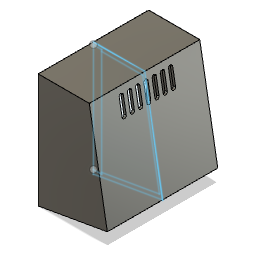
TrafficLight (Autodesk Fusion 360 archive; units mm, degrees)
design "PraxisAmpel2"
Autodesk Fusion 360 part; units mm, degrees
sketch "Sketch1" plane through (0, 0, 0) normal (0, 0, 1) x (1, 0, 0)
  line L0 (7.1104, -4.3777) -> (49.1586, 3.0365)
  line L1 (49.1586, 3.0365) -> (38.1927, 65.227)
  line L2 (38.1927, 65.227) -> (7.1104, 65.227)
  line L3 (7.1104, 65.227) -> (7.1104, -4.3777)
  line L4 (7.1104, 63.727) -> (12.1104, 63.727)
  line L5 (12.1104, 63.727) -> (12.1104, -1.973)
  line L6 (12.1104, -1.973) -> (7.1104, -1.973)
  line L7 (12.1104, 62.727) -> (37.1104, 62.727)
  line L8 (37.1104, 62.727) -> (47.2499, 5.2231)
  line L9 (47.2499, 5.2231) -> (12.1104, -0.973)
  dimension "d5" = 80
  dimension "d6" = 1.5
  dimension "d8" = 5
  dimension "d9" = 65.7
  dimension "d11" = 1.5
  dimension "d12" = 1
  dimension "d13" = 1
  dimension "d40" = 1.5
  dimension "d41" = 30
  constraint horizontal L2
  constraint vertical L3
  constraint perpendicular L0 L1
  constraint horizontal L4
  constraint vertical L5
  constraint horizontal L6
  constraint coincident L3 L4.start
  constraint coincident L5 L7.start
  constraint perpendicular L5 L7
  constraint parallel L1 L8
  constraint coincident L5 L9.end
  constraint parallel L0 L9
  measures "d5" angle of L0 L3
  measures "d6" distance of L2 L4
  measures "d8" distance of L3 L5
  measures "d9" distance of L4 L6
  measures "d11" distance of L0 L5.end
  measures "d12" distance of L5.end L9.end
  measures "d13" distance of L4.end L7.start
  measures "d40" distance of L1 L8
  measures "d41" horizontal distance of L4.start L7.end
extrude "Extrude4" add sketch "Sketch1" against normal blind 32.1 contours L3 L4 L5 L6 | L5 L7 L8 L9 makes body 1
extrude "Extrude3" add sketch "Sketch1" along normal blind 32.1 separate body contours L3 L4 L5 L6 | L5 L7 L8 L9 makes body 2
extrude "Extrude1" add sketch "Sketch1" along normal blind 33.6 separate body makes body 3
extrude "Extrude2" add 1 faces at (31.4873, 22.0968, 0) along direction (0, 0, -1) blind 33.6 on bodies 3 bodies 3
combine "Combine1" operation add target body 1 tool bodies 2
combine "Combine2" operation cut target body 3 tool bodies 1
sketch "Sketch2" plane through (0, 0, -33.6) normal (0, 0, -1) x (-1, 0, 0)
  line L0 (-7.1104, -4.3777) -> (-7.1104, 65.227)
  line L1 (-7.1104, 65.227) -> (-38.1927, 65.227)
  line L2 (-38.1927, 65.227) -> (-49.1586, 3.0365)
  line L3 (-49.1586, 3.0365) -> (-7.1104, -4.3777)
  line L4 (-7.1104, 8.6223) -> (-15.1104, 8.6223)
  line L5 (-17.1104, 6.6223) -> (-17.1104, 5.6223)
  line L6 (-15.1104, 3.6223) -> (-7.1104, 3.6223)
  arc A0 (-15.1104, 8.6223) -> (-17.1104, 6.6223) centre (-15.1104, 6.6223) ccw
  arc A1 (-17.1104, 5.6223) -> (-15.1104, 3.6223) centre (-15.1104, 5.6223) ccw
  line L7 (-7.1104, 65.227) -> (-7.1104, -4.3777)
  dimension "d23" = 2
  dimension "d24" = 2
  dimension "d26" = 8
  dimension "d27" = 10
  dimension "d28" = 5
  constraint coincident L0 L4.start
  constraint perpendicular L0 L4
  constraint perpendicular L4 L5
  constraint perpendicular L0 L6
  constraint tangent L4 A0
  constraint tangent L5 A0
  constraint tangent L5 A1
  constraint tangent L6 A1
  measures "d23" radius of A0
  measures "d24" radius of A1
  measures "d26" distance of L0.start L6
  measures "d27" distance of L5 L7
  measures "d28" distance of L4 L6
extrude "Extrude5" cut sketch "Sketch2" against normal blind 1.5 contours L0 L4 L5 L6 A0 A1 L7 bodies 3
sketch "Sketch3" plane through (48.1956, 8.4982, 0) normal (0.984808, 0.173648, 0) x (0, 0, -1)
  line L0 (33.6, 57.604) -> (-33.6, 57.604)
  line L1 (-33.6, 57.604) -> (-33.6, -5.546)
  line L2 (-33.6, -5.546) -> (33.6, -5.546)
  line L3 (33.6, -5.546) -> (33.6, 57.604)
  line L4 (1.25, 42.604) -> (1.25, 52.604)
  arc A0 (1.25, 52.604) -> (-1.25, 52.604) centre (0, 52.604) ccw
  line L5 (-1.25, 52.604) -> (-1.25, 42.604)
  arc A1 (-1.25, 42.604) -> (1.25, 42.604) centre (0, 42.604) ccw
  line L6 (0, 42.604) -> (0, 52.604) construction
  line L7 (0, 57.604) -> (0, 47.604) construction
  arc A2 (-13.75, 52.604) -> (-16.25, 52.604) centre (-15, 52.604) ccw
  arc A3 (-16.25, 42.604) -> (-13.75, 42.604) centre (-15, 42.604) ccw
  line L8 (-13.75, 42.604) -> (-13.75, 52.604)
  line L9 (-16.25, 52.604) -> (-16.25, 42.604)
  arc A4 (-8.75, 52.604) -> (-11.25, 52.604) centre (-10, 52.604) ccw
  arc A5 (-11.25, 42.604) -> (-8.75, 42.604) centre (-10, 42.604) ccw
  line L10 (-8.75, 42.604) -> (-8.75, 52.604)
  line L11 (-11.25, 52.604) -> (-11.25, 42.604)
  arc A6 (-3.75, 52.604) -> (-6.25, 52.604) centre (-5, 52.604) ccw
  arc A7 (-6.25, 42.604) -> (-3.75, 42.604) centre (-5, 42.604) ccw
  line L12 (-3.75, 42.604) -> (-3.75, 52.604)
  line L13 (-6.25, 52.604) -> (-6.25, 42.604)
  arc A8 (6.25, 52.604) -> (3.75, 52.604) centre (5, 52.604) ccw
  arc A9 (3.75, 42.604) -> (6.25, 42.604) centre (5, 42.604) ccw
  line L14 (6.25, 42.604) -> (6.25, 52.604)
  line L15 (3.75, 52.604) -> (3.75, 42.604)
  arc A10 (11.25, 52.604) -> (8.75, 52.604) centre (10, 52.604) ccw
  arc A11 (8.75, 42.604) -> (11.25, 42.604) centre (10, 42.604) ccw
  line L16 (11.25, 42.604) -> (11.25, 52.604)
  line L17 (8.75, 52.604) -> (8.75, 42.604)
  arc A12 (16.25, 52.604) -> (13.75, 52.604) centre (15, 52.604) ccw
  arc A13 (13.75, 42.604) -> (16.25, 42.604) centre (15, 42.604) ccw
  line L18 (16.25, 42.604) -> (16.25, 52.604)
  line L19 (13.75, 52.604) -> (13.75, 42.604)
  point P0 (0, 47.604)
  dimension "d31" = 2.5
  dimension "d32" = 10
  dimension "d33" = 10
  dimension "d36" = 5
  dimension "d37" = 0
  constraint tangent L4 A0
  constraint tangent A0 L5
  constraint parallel L4 L5
  constraint tangent L5 A1
  constraint tangent L4 A1
  constraint vertical L6
  constraint midpoint L6 P0
  constraint midpoint L0 L7.start
  constraint perpendicular L0 L7
  constraint coincident P0 L7.end
  measures "d31" diameter of A0
  measures "d32" distance of A1.centre A0.centre
  measures "d33" distance of L7.start P0
extrude "Extrude6" cut sketch "Sketch3" against normal blind 1.5 contours L4 A0 L5 A1 | A2 A3 L8 L9 | A4 A5 L10 L11 | A6 A7 L12 L13 | A8 A9 L14 L15 | A10 A11 L16 L17 | A12 A13 L18 L19 bodies 3
equation "wall_thickness = 1.5 mm"
equation "d6 = wall_thickness"
equation "d9 = 64.2 mm + wall_thickness"
equation "d11 = wall_thickness"
equation "d14 = 32.1 mm + wall_thickness"
equation "d16 = 32.1 mm + wall_thickness"
equation "d29 = -wall_thickness"
equation "d38 = -wall_thickness"
equation "d40 = wall_thickness"
